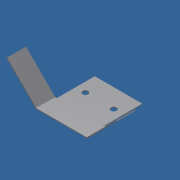
# Autodesk Inventor part: PÁRA LAMA TRASEIRO
Saved by Autodesk Inventor 2012 SP1 (Build 160190100, 190)
## iProperties
Created: 2012-07-23
Part Number: PÁRA LAMA TRASEIRO
Material: Default
Document SubType Name: Sheet Metal
Designer: bruno.silveira
Density: 1 g/cm^3
Sheet Metal Rule: Default
Author: bruno.silveira
Autodesk Inventor part; units mm, degrees
ref_plane "YZ Plane" through (0, 0, 0) normal (1, 0, 0) x (0, 1, 0)
ref_plane "XZ Plane" through (0, 0, 0) normal (0, 1, 0) x (-1, 0, 0)
ref_plane "XY Plane" through (0, 0, 0) normal (0, 0, 1) x (1, 0, 0)
sketch "Sketch1" plane through (0, 0, 0) normal (0, 0, 1) x (1, 0, 0)
  line L0 (0, 0) -> (0, 10)
  line L1 (0, 10) -> (21, 10)
  line L2 (22, 10) -> (22, 30)
  line L3 (22, 30) -> (47, 30)
  line L4 (47, 30) -> (47, 10)
  line L5 (48, 10) -> (69, 10)
  line L6 (69, 10) -> (69, 0)
  line L7 (21, 10) -> (21, 0)
  line L8 (48, 10) -> (48, 0)
  line L9 (69, 0) -> (48, 0)
  line L10 (21, 0) -> (0, 0)
  line L11 (21, 0) -> (48, 0)
  line L12 (48, 10) -> (47, 10)
  line L13 (21, 10) -> (22, 10)
  dimension "d0" = 22
  dimension "d1" = 22
  dimension "d2" = 10
  dimension "d3" = 25
  dimension "d5" = 10
  dimension "d8" = 1
  dimension "d9" = 1
  measures "d0" distance of L0.end L2.start
  measures "d1" distance of L4.end L5.end
  measures "d2" distance of L0.start L0.end
  measures "d3" distance of L2.end L3.end
  measures "d5" distance of L5.end L6.end
  measures "d8" distance between parallel lines of L2 L7
  measures "d9" distance between parallel lines of L4 L8
extrude "Plate1" add sketch "Sketch1" along normal blind 0.5 contours L7 L13 L2 L3 L4 L12 L8 L11
sketch "Sketch2" plane through (21.3536, 0, 0.3536) normal (-0.7071068, 0, -0.7071068) x (0, -1, 0)
  line L0 (-10, 0) -> (0, 0)
  line L1 (0, 0) -> (0, 22)
  line L2 (0, 22) -> (-10, 22)
  line L3 (-10, 22) -> (-10, 0)
  constraints: 4 end point, 4 other
edge flange "Flange1" height 22 angle 45 thickness 0.5 bend radius 0.5 thickness toward (-0.7071068, 0, -0.7071068) relief straight relief width 0.5 relief depth 0.25 corner gap 0.5 corner form 0 edges at (21, 5, 0.5) (48, 5, 0.5) wall of the first edge with corners at (21.3536, 10, 0.3536) (21.3536, 0, 0.3536) (5.7972, 0, 15.9099) (5.7972, 10, 15.9099)
bend "Bend1"
corner "Corner1"
sketch "Sketch3" plane through (0, 0, 0) normal (0, 0, -1) x (-1, 0, 0)
  line L0 (-21.4142, 0) -> (-47.5858, 0) projected
  line L1 (-47, 10) -> (-47, 30) projected
  circle A0 centre (-42, 20) radius 1.5
  circle A1 centre (-27, 20) radius 1.5
  point P0 (0, 0)
  dimension "d21" = 3
  dimension "d22" = 3
  dimension "d23" = 15
  dimension "d24" = 20
  dimension "d25" = 5
  constraints: 2 centre point
  measures "d21" diameter of A1
  measures "d22" diameter of A0
  measures "d23" distance of A1.centre A0.centre
  measures "d24" distance from line of L0 A1.centre
  measures "d25" distance from line of L1 A0.centre
hole "Hole1" at (42, 20, 0) at (27, 20, 0) direction (0, 0, 1) diameter 3 depth 0.5 tip angle 118
equation "\"d31\" = Thickness"
equation "\"d11\" = BendReliefWidth"
equation "\"d12\" = BendReliefDepth"
equation "\"d13\" = MinimumRemnant"
equation "\"d14\" = BendRadius"
equation "\"d17\" = BendRadius"
equation "\"d18\" = CornerReliefSize"
equation "\"d19\" = GapSize"
equation "\"d20\" = JacobiRadiusSize"
equation "\"BendRadius\" = Thickness"
equation "\"BendReliefWidth\" = Thickness"
equation "\"BendReliefDepth\" = 0.5 * Thickness"
equation "\"CornerReliefSize\" = 4 * Thickness"
equation "\"MinimumRemnant\" = 2 * Thickness"
equation "\"TransitionRadius\" = BendRadius"
equation "\"JacobiRadiusSize\" = Thickness"
equation "\"GapSize\" = Thickness"
equation "\"d10\" = BendRadius"
equation "\"Thickness\" = 0.5"
body "Solid1"
